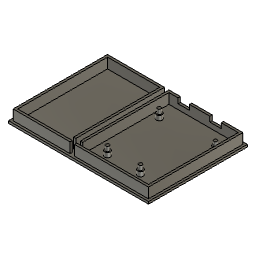
3dModel (Autodesk Fusion 360 design; units mm, degrees)
Autodesk Fusion 360 part; units mm, degrees
sketch "Sketch1" plane through (0, 0, 0) normal (0, 0, 1) x (1, 0, 0)
  line L0 (-88.4927, 61.808) -> (34.5073, 61.808)
  line L1 (34.5073, 61.808) -> (34.5073, -25.192)
  line L2 (34.5073, -25.192) -> (-88.4927, -25.192)
  line L3 (-88.4927, -25.192) -> (-88.4927, 61.808)
  dimension "d1" = 123
  dimension "d2" = 87
  constraint horizontal L0
  constraint vertical L1
  constraint horizontal L2
  constraint vertical L3
  measures "d1" distance of L0.start L0.end
  measures "d2" distance of L0.start L2.end
extrude "Extrude1" add sketch "Sketch1" along normal blind 2
sketch "Sketch2" plane through (0, 0, 2) normal (0, 0, 1) x (-1, 0, 0)
  line L0 (88.4927, 25.192) -> (-34.5073, 25.192)
  line L1 (-34.5073, 25.192) -> (-34.5073, -61.808)
  line L2 (-34.5073, -61.808) -> (88.4927, -61.808)
  line L3 (88.4927, -61.808) -> (88.4927, 25.192)
  line L4 (88.4927, -61.808) -> (88.4927, -59.808)
  line L5 (88.4927, -61.808) -> (86.4927, -61.808)
  line L6 (86.4927, -61.808) -> (86.4927, -59.808)
  line L7 (86.4927, -59.808) -> (36.4927, -59.808)
  line L8 (88.4927, 25.192) -> (86.4927, 25.192)
  line L9 (86.4927, -59.808) -> (86.4927, 23.192)
  line L10 (86.4927, 23.192) -> (36.4927, 23.192)
  line L11 (86.4927, -59.808) -> (84.4927, -59.808)
  line L12 (36.4927, 23.192) -> (36.4927, 21.192)
  line L13 (36.4927, 21.192) -> (38.4927, 21.192)
  line L14 (84.4927, -57.808) -> (38.4927, -57.808)
  line L15 (38.4927, -57.808) -> (38.4927, 18.0206)
  line L16 (38.4927, 21.192) -> (84.4927, 21.192)
  line L17 (84.4927, 21.192) -> (84.4927, -57.808)
  line L18 (38.4927, 18.0206) -> (36.4927, 18.0206)
  line L19 (36.4927, -59.808) -> (36.4927, 18.0206)
  line L20 (36.4927, 21.192) -> (36.4927, 23.192)
  line L21 (-34.5073, 25.192) -> (-34.5073, 23.192)
  line L22 (-34.5073, 23.192) -> (-32.5073, 23.192)
  line L23 (-32.5073, -59.808) -> (-32.5073, 23.192)
  line L24 (-32.5073, 23.192) -> (32.4927, 23.192)
  line L25 (32.4927, -59.808) -> (30.4927, -59.808)
  line L26 (-32.5073, 23.192) -> (-32.5073, 21.192)
  line L27 (-30.5073, -57.808) -> (-30.5073, 21.192)
  line L28 (-30.5073, 21.192) -> (30.4927, 21.192)
  line L29 (30.4927, 18.0206) -> (30.4927, -57.808)
  line L30 (32.4927, 18.0206) -> (30.4927, 18.0206)
  line L31 (30.4927, 21.192) -> (32.4927, 21.192)
  line L32 (32.4927, 23.192) -> (32.4927, 21.192)
  line L33 (32.4927, 18.0206) -> (32.4927, -59.808)
  line L34 (30.4927, -59.808) -> (22.4927, -59.808)
  line L35 (12.4927, -59.808) -> (12.4927, -57.808)
  line L36 (22.4927, -57.808) -> (22.4927, -59.808)
  line L37 (30.4927, -57.808) -> (22.4927, -57.808)
  line L38 (32.4927, -59.808) -> (22.4927, -59.808)
  line L39 (12.4927, -59.808) -> (-32.5073, -59.808)
  line L40 (-32.5073, -59.808) -> (-15.5073, -59.808)
  line L41 (-5.5073, -59.808) -> (-5.5073, -57.808)
  line L42 (-5.5073, -57.808) -> (-15.5073, -57.808)
  line L43 (-15.5073, -57.808) -> (-15.5073, -59.808)
  line L44 (12.4927, -57.808) -> (-5.5073, -57.808)
  line L45 (-15.5073, -57.808) -> (-30.5073, -57.808)
  dimension "d5" = 2
  dimension "d6" = 2
  dimension "d7" = 2
  dimension "d8" = 50
  dimension "d9" = 2
  dimension "d10" = 2
  dimension "d11" = 50
  dimension "d12" = 2
  dimension "d13" = 2
  dimension "d14" = 2
  dimension "d15" = 2
  dimension "d17" = 4
  dimension "d18" = 2
  dimension "d19" = 2
  dimension "d20" = 2
  dimension "d21" = 2
  dimension "d22" = 2
  dimension "d23" = 2
  dimension "d24" = 8
  dimension "d25" = 10
  dimension "d26" = 17
  dimension "d27" = 10
  constraint coincident L2.end L3.start
  constraint perpendicular L2 L4
  constraint perpendicular L3 L5
  constraint perpendicular L5 L6
  constraint perpendicular L6 L7
  constraint coincident L0.start L3.end
  constraint perpendicular L3 L8
  constraint perpendicular L9 L10
  constraint perpendicular L9 L11
  constraint perpendicular L10 L12
  constraint perpendicular L13 L19
  constraint horizontal L14
  constraint vertical L15
  constraint horizontal L16
  constraint vertical L17
  constraint perpendicular L18 L19
  constraint collinear L19 L20
  constraint coincident L0.end L1.start
  constraint perpendicular L0 L21
  constraint perpendicular L1 L22
  constraint horizontal L38
  constraint vertical L23
  constraint horizontal L24
  constraint vertical L32
  constraint perpendicular L25 L32
  constraint perpendicular L24 L26
  constraint horizontal L37
  constraint vertical L27
  constraint horizontal L28
  constraint vertical L29
  constraint perpendicular L29 L30
  constraint perpendicular L20 L31
  constraint collinear L32 L33
  constraint parallel L34 L38
  constraint vertical L35
  constraint vertical L36
  constraint collinear L37 L44
  constraint collinear L38 L39
  constraint perpendicular L23 L40
  constraint vertical L41
  constraint horizontal L42
  constraint vertical L43
  constraint collinear L44 L45
  measures "d5" distance of L2.end L4.end
  measures "d6" distance of L2.end L5.end
  measures "d7" distance of L5.end L6.end
  measures "d8" distance of L6.end L7.end
  measures "d9" distance of L0.start L8.end
  measures "d10" distance of L8.end L9.end
  measures "d11" distance of L9.end L10.end
  measures "d12" distance of L6.end L11.end
  measures "d13" distance of L11.end L14.start
  measures "d14" distance of L10.end L12.end
  measures "d15" distance of L12.end L13.end
  measures "d17" distance of L7.end L25.start
  measures "d18" distance of L0.end L21.end
  measures "d19" distance of L21.end L22.end
  measures "d20" distance of L25.start L25.end
  measures "d21" distance of L25.end L29.end
  measures "d22" distance of L22.end L26.end
  measures "d23" distance of L26.end L27.end
  measures "d24" distance of L25.end L34.end
  measures "d25" distance of L34.end L35.start
  measures "d26" distance of L23.start L40.end
  measures "d27" distance of L40.end L41.start
extrude "Extrude2" add sketch "Sketch2" along normal blind 9 contours L7 L9 L10 L11 L12 L13 L14 L15 L16 L17 L18 L19 L20 | L23 L24 L26 L27 L28 L31 L32 L39 L40 L43 L45 | L35 L39 L41 L44 | L25 L29 L30 L33 L34 L36 L37 L38
sketch "Sketch3" plane through (0, 0, 2) normal (0, 0, 1) x (-1, 0, 0)
  line L0 (12.4927, -59.808) -> (-5.5073, -59.808)
  line L1 (-5.5073, -59.808) -> (-5.5073, -57.808)
  line L2 (-5.5073, -57.808) -> (12.4927, -57.808)
  line L3 (12.4927, -57.808) -> (12.4927, -59.808)
  line L4 (36.4927, 21.192) -> (36.4927, 23.192)
  line L5 (36.4927, 23.192) -> (86.4927, 23.192)
  line L6 (86.4927, 23.192) -> (86.4927, -59.808)
  line L7 (86.4927, -59.808) -> (36.4927, -59.808)
  line L8 (36.4927, -59.808) -> (36.4927, 18.0206)
  line L9 (36.4927, 18.0206) -> (38.4927, 18.0206)
  line L10 (38.4927, 18.0206) -> (38.4927, -57.808)
  line L11 (38.4927, -57.808) -> (84.4927, -57.808)
  line L12 (84.4927, -57.808) -> (84.4927, 21.192)
  line L13 (84.4927, 21.192) -> (36.4927, 21.192)
  line L14 (-32.5073, -59.808) -> (-32.5073, 23.192)
  line L15 (-32.5073, 23.192) -> (32.4927, 23.192)
  line L16 (32.4927, 23.192) -> (32.4927, 21.192)
  line L17 (32.4927, 21.192) -> (-30.5073, 21.192)
  line L18 (-30.5073, 21.192) -> (-30.5073, -57.808)
  line L19 (-30.5073, -57.808) -> (-15.5073, -57.808)
  line L20 (-15.5073, -57.808) -> (-15.5073, -59.808)
  line L21 (-15.5073, -59.808) -> (-32.5073, -59.808)
  line L22 (32.4927, 18.0206) -> (32.4927, -59.808)
  line L23 (32.4927, -59.808) -> (22.4927, -59.808)
  line L24 (22.4927, -59.808) -> (22.4927, -57.808)
  line L25 (22.4927, -57.808) -> (30.4927, -57.808)
  line L26 (30.4927, -57.808) -> (30.4927, 18.0206)
  line L27 (30.4927, 18.0206) -> (32.4927, 18.0206)
  line L28 (88.4927, 25.192) -> (-34.5073, 25.192)
  line L29 (-34.5073, 25.192) -> (-34.5073, -61.808)
  line L30 (-34.5073, -61.808) -> (88.4927, -61.808)
  line L31 (88.4927, -61.808) -> (88.4927, 25.192)
  line L32 (-5.5073, -59.808) -> (-15.5073, -59.808)
  line L33 (-15.5073, -59.808) -> (-15.5073, -57.808)
  line L34 (-15.5073, -57.808) -> (-5.5073, -57.808)
  line L35 (-5.5073, -57.808) -> (-5.5073, -59.808)
  constraint horizontal L32
  constraint vertical L33
  constraint horizontal L34
  constraint vertical L35
  constraint coincident L19.end L20.start
  constraint coincident L0.end L1.start
extrude "Extrude3" add sketch "Sketch3" along normal blind 4.5 contours L1 L20 L32 L33 L34 L35
sketch "Sketch4" plane through (0, 0, 2) normal (0, 0, 1) x (-1, 0, 0)
  line L0 (88.4927, 25.192) -> (-34.5073, 25.192)
  line L1 (-34.5073, 25.192) -> (-34.5073, -61.808)
  line L2 (-34.5073, -61.808) -> (88.4927, -61.808)
  line L3 (88.4927, -61.808) -> (88.4927, 25.192)
  line L4 (32.4927, 18.0206) -> (32.4927, -59.808)
  line L5 (32.4927, -59.808) -> (22.4927, -59.808)
  line L6 (22.4927, -59.808) -> (22.4927, -57.808)
  line L7 (22.4927, -57.808) -> (30.4927, -57.808)
  line L8 (30.4927, -57.808) -> (30.4927, 18.0206)
  line L9 (30.4927, 18.0206) -> (32.4927, 18.0206)
  line L10 (12.4927, -59.808) -> (-32.5073, -59.808)
  line L11 (-32.5073, -59.808) -> (-32.5073, 23.192)
  line L12 (-32.5073, 23.192) -> (32.4927, 23.192)
  line L13 (32.4927, 23.192) -> (32.4927, 21.192)
  line L14 (32.4927, 21.192) -> (-30.5073, 21.192)
  line L15 (-30.5073, 21.192) -> (-30.5073, -57.808)
  line L16 (-30.5073, -57.808) -> (12.4927, -57.808)
  line L17 (12.4927, -57.808) -> (12.4927, -59.808)
  line L18 (36.4927, 21.192) -> (36.4927, 23.192)
  line L19 (36.4927, 23.192) -> (86.4927, 23.192)
  line L20 (86.4927, 23.192) -> (86.4927, -59.808)
  line L21 (86.4927, -59.808) -> (36.4927, -59.808)
  line L22 (36.4927, -59.808) -> (36.4927, 18.0206)
  line L23 (36.4927, 18.0206) -> (38.4927, 18.0206)
  line L24 (38.4927, 18.0206) -> (38.4927, -57.808)
  line L25 (38.4927, -57.808) -> (84.4927, -57.808)
  line L26 (84.4927, -57.808) -> (84.4927, 21.192)
  line L27 (84.4927, 21.192) -> (36.4927, 21.192)
  circle A0 centre (23.9927, -42.808) radius 2.5
  circle A1 centre (-25.5073, -42.808) radius 2.5
  circle A2 centre (-10.5073, 8.192) radius 2.5
  circle A3 centre (18.4927, 8.192) radius 2.5
  dimension "d34" = 5
  dimension "d36" = 5
  dimension "d39" = 5
  dimension "d41" = 5
  measures "d34" diameter of A0
  measures "d36" diameter of A1
  measures "d39" diameter of A2
  measures "d41" diameter of A3
extrude "Extrude4" add sketch "Sketch4" along normal blind 4 contours A0 | A1 | A2 | A3
sketch "Sketch5" plane through (0, 0, 6) normal (0, 0, 1) x (-1, 0, 0)
  circle A0 centre (23.9927, -42.808) radius 2.5
  circle A1 centre (23.9927, -42.808) radius 1.5
  dimension "d44" = 3
  constraint concentric A0 A1
  measures "d44" diameter of A1
extrude "Extrude5" add sketch "Sketch5" along normal blind 4 contours A1
sketch "Sketch6" plane through (0, 0, 6) normal (0, 0, 1) x (-1, 0, 0)
  circle A0 centre (-25.5073, -42.808) radius 2.5
  circle A1 centre (-25.5073, -42.808) radius 1.5
  dimension "d47" = 3
  constraint concentric A0 A1
  measures "d47" diameter of A1
extrude "Extrude6" add sketch "Sketch6" along normal blind 4 contours A1
sketch "Sketch7" plane through (0, 0, 6) normal (0, 0, 1) x (-1, 0, 0)
  circle A0 centre (18.4927, 8.192) radius 2.5
  circle A1 centre (18.4927, 8.192) radius 1.5
  dimension "d50" = 3
  constraint concentric A0 A1
  measures "d50" diameter of A1
extrude "Extrude7" add sketch "Sketch7" along normal blind 4 contours A1
sketch "Sketch8" plane through (0, 0, 6) normal (0, 0, 1) x (-1, 0, 0)
  circle A0 centre (-10.5073, 8.192) radius 2.5
  circle A1 centre (-10.5073, 8.192) radius 1.5
  dimension "d53" = 3
  constraint concentric A0 A1
  measures "d53" diameter of A1
extrude "Extrude8" add sketch "Sketch8" along normal blind 4 contours A1
sketch "Sketch9" plane through (0, 0, 2) normal (0, 0, 1) x (-1, 0, 0)
  circle A0 centre (18.4927, 8.192) radius 2.5
  circle A1 centre (23.9927, -42.808) radius 2.5
  circle A2 centre (-10.5073, 8.192) radius 2.5
  circle A3 centre (-25.5073, -42.808) radius 2.5
  line L0 (88.4927, 25.192) -> (-34.5073, 25.192)
  line L1 (-34.5073, 25.192) -> (-34.5073, -61.808)
  line L2 (-34.5073, -61.808) -> (88.4927, -61.808)
  line L3 (88.4927, -61.808) -> (88.4927, 25.192)
  line L4 (32.4927, 18.0206) -> (32.4927, -59.808)
  line L5 (32.4927, -59.808) -> (22.4927, -59.808)
  line L6 (22.4927, -59.808) -> (22.4927, -57.808)
  line L7 (22.4927, -57.808) -> (30.4927, -57.808)
  line L8 (30.4927, -57.808) -> (30.4927, 18.0206)
  line L9 (30.4927, 18.0206) -> (32.4927, 18.0206)
  line L10 (12.4927, -59.808) -> (-32.5073, -59.808)
  line L11 (-32.5073, -59.808) -> (-32.5073, 23.192)
  line L12 (-32.5073, 23.192) -> (32.4927, 23.192)
  line L13 (32.4927, 23.192) -> (32.4927, 21.192)
  line L14 (32.4927, 21.192) -> (-30.5073, 21.192)
  line L15 (-30.5073, 21.192) -> (-30.5073, -57.808)
  line L16 (-30.5073, -57.808) -> (12.4927, -57.808)
  line L17 (12.4927, -57.808) -> (12.4927, -59.808)
  line L18 (36.4927, 21.192) -> (36.4927, 23.192)
  line L19 (36.4927, 23.192) -> (86.4927, 23.192)
  line L20 (86.4927, 23.192) -> (86.4927, -59.808)
  line L21 (86.4927, -59.808) -> (36.4927, -59.808)
  line L22 (36.4927, -59.808) -> (36.4927, 18.0206)
  line L23 (36.4927, 18.0206) -> (38.4927, 18.0206)
  line L24 (38.4927, 18.0206) -> (38.4927, -57.808)
  line L25 (38.4927, -57.808) -> (84.4927, -57.808)
  line L26 (84.4927, -57.808) -> (84.4927, 21.192)
  line L27 (84.4927, 21.192) -> (36.4927, 21.192)
  line L28 (22.4927, -59.808) -> (12.4927, -59.808)
  line L29 (12.4927, -59.808) -> (12.4927, -57.808)
  line L30 (12.4927, -57.808) -> (22.4927, -57.808)
  line L31 (22.4927, -57.808) -> (22.4927, -59.808)
  constraint horizontal L28
  constraint vertical L29
  constraint horizontal L30
  constraint vertical L31
  constraint coincident L16.end L17.start
  constraint coincident L5.end L6.start
extrude "Extrude9" add sketch "Sketch9" along normal blind 4.5 contours L6 L17 L28 L29 L30 L31
